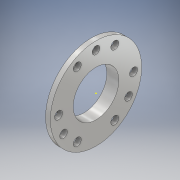
# Autodesk Inventor part: Cathode Holder Cap
Saved by Autodesk Inventor 2017.3 (Build 213256000, 256)
## iProperties
Created: 2017-02-02
Part Number: Cathode Holder Cap
Material: Generic
Document SubType Name: Modeling
Designer: Mac
Density: 1 g/cm^3
Appearance: Aluminum - Dark
Author: Mac
Autodesk Inventor part; units mm, degrees
ref_plane "YZ Plane" through (0, 0, 0) normal (1, 0, 0) x (0, 1, 0)
ref_plane "XZ Plane" through (0, 0, 0) normal (0, 1, 0) x (-1, 0, 0)
ref_plane "XY Plane" through (0, 0, 0) normal (0, 0, 1) x (1, 0, 0)
sketch "Sketch1" plane through (0, 0, 0) normal (1, 0, 0) x (0, 1, 0)
  circle A0 centre (0, 0) radius 9.5
  dimension "d0" = 19
  constraints: 1 centre point, 1 coincident
  measures "d0" diameter of A0
extrude "Extrusion1" add sketch "Sketch1" along normal blind 1
sketch "Sketch2" plane through (1, 0, 0) normal (1, 0, 0) x (0, 0, -1)
  circle A0 centre (0, 0) radius 0.5
  circle A1 centre (0, 7.81) radius 0.835
  circle A2 centre (0, -7.81) radius 0.835
  circle A3 centre (6.7637, 3.905) radius 0.835
  circle A4 centre (6.7637, -3.905) radius 0.835
  circle A5 centre (-6.7637, -3.905) radius 0.835
  circle A6 centre (-6.7637, 3.905) radius 0.835
  dimension "d3" = 1
  dimension "d4" = 1.67
  dimension "d5" = 1.67
  dimension "d6" = 1.67
  dimension "d7" = 1.67
  dimension "d8" = 1.67
  dimension "d9" = 1.67
  constraints: 7 centre point, 1 coincident
  measures "d3" diameter of A0
  measures "d4" diameter of A1
  measures "d5" diameter of A2
  measures "d6" diameter of A3
  measures "d7" diameter of A4
  measures "d8" diameter of A5
  measures "d9" diameter of A6
sketch "Sketch3" plane through (0, 0, 0) normal (-1, 0, 0) x (0, 0, 1)
  circle A0 centre (0, 0) radius 6
  dimension "d10" = 12
  constraints: 1 centre point, 1 coincident
  measures "d10" diameter of A0
extrude "Extrusion2" add sketch "Sketch3" along normal blind 1.5
extrude "Extrusion3" cut sketch "Sketch2" against normal blind 1 contours A1 | A2 | A3 | A4 | A5 | A6
sketch "Sketch4" plane through (1, 0, 0) normal (1, 0, 0) x (0, 0, -1)
  point P0 (0, 0)
ref_plane "Work Plane1" through (1, 0, 0) normal (1, 0, 0) x (0, 0, -1)
ref_plane "Work Plane2" through (1, 3.905, 6.7637) normal (0, 0, 1) x (-1, 0, 0)
sketch "Sketch5" plane through (1, 0, 0) normal (1, 0, 0) x (0, 0, -1)
  point P0 (0, 0)
sketch "Sketch6" plane through (1, 0, 0) normal (1, 0, 0) x (0, 0, -1)
  point P0 (0, 0)
sketch "Sketch7" plane through (1, 0, 0) normal (1, 0, 0) x (0, 0, -1)
  point P0 (0, 0)
sketch "Sketch8" plane through (1, 0, 0) normal (1, 0, 0) x (0, 0, -1)
  point P0 (0, 0)
  point P1 (-7.81, 0)
  point P2 (3.905, 6.7637)
  point P3 (3.905, -6.764)
hole "Hole1" at (1, 0, 7.81) at (1, -6.764, -3.905) at (1, 6.7637, -3.905) direction (-1, 0, 0) diameter 1.6 depth 1
sketch "Sketch9" plane through (-1.5, 0, 0) normal (-1, 0, 0) x (0, 0, 1)
  circle A0 centre (0, 0) radius 4.75
  dimension "d23" = 9.5
  constraints: 1 centre point, 1 coincident
  measures "d23" diameter of A0
extrude "Extrusion4" cut sketch "Sketch9" against normal blind 3
body "Solid1"
